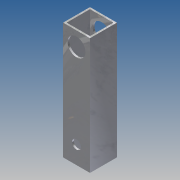
# Autodesk Inventor part: Z_Stage_Nut_holder_15x15alu
Saved by Autodesk Inventor 2015 SP1 (Build 190203100, 203)
## iProperties
Created: 2015-03-05
Part Number: Z_Stage_Nut_holder_15x15alu
Material: Aluminium 6061
Document SubType Name: Modeling
Designer: Marc
Density: 2.7 g/cm^3
Appearance: Aluminium - flach
Mass: 9.29786 g
Surface Area: 70.9355 cm^2
Volume: 3.44365 cm^3
Author: Marc
Autodesk Inventor part; units mm, degrees
ref_plane "YZ Plane" through (0, 0, 0) normal (1, 0, 0) x (0, 1, 0)
ref_plane "XZ Plane" through (0, 0, 0) normal (0, 1, 0) x (-1, 0, 0)
ref_plane "XY Plane" through (0, 0, 0) normal (0, 0, 1) x (1, 0, 0)
sketch "Skizze1" plane through (0, 0, 0) normal (0, 0, 1) x (1, 0, 0)
  line L0 (-10.5, 0) -> (10.5, 0) projected
  line L1 (0, -10.5) -> (0, 10.5) projected
  line L2 (-7.5, -7.5) -> (7.5, -7.5)
  line L3 (7.5, -7.5) -> (7.5, 7.5)
  line L4 (7.5, 7.5) -> (-7.5, 7.5)
  line L5 (-7.5, 7.5) -> (-7.5, -7.5)
  line L6 (-6.5, -6.5) -> (6.5, -6.5)
  line L7 (6.5, -6.5) -> (6.5, 6.5)
  line L8 (6.5, 6.5) -> (-6.5, 6.5)
  line L9 (-6.5, 6.5) -> (-6.5, -6.5)
  line L10 (-6.5, -6.5) -> (6.5, 6.5) construction
  line L11 (6.5, -6.5) -> (-6.5, 6.5) construction
  point P0 (0, 0)
  dimension "d0" = 15
  dimension "d1" = 15
  dimension "d2" = 13
  dimension "d3" = 13
  constraints: 20 end point, 4 parallel, 2 horizontal, 2 midpoint, 2 perpendicular, 2 other
  measures "d0" distance of L4.end L3.end
  measures "d1" distance of L3.end L2.end
  measures "d2" distance of L8.end L7.end
  measures "d3" distance of L7.end L6.end
extrude "Extrusion1" add sketch "Skizze1" along normal blind 65 contours L5 L4 L1 L8 L9 L0 | L0 L9 L6 L1 L2 L5 | L4 L3 L0 L7 L8 L1 | L1 L6 L7 L0 L3 L2
sketch "Skizze2" plane through (-7.5, 7.5, 0) normal (0, 1, 0) x (1, 0, 0)
  line L0 (15, 0) -> (0, 0) projected
  line L1 (0, 0) -> (0, -65) projected
  line L2 (15, -65) -> (0, -65) projected
  line L3 (15, 0) -> (15, -65) projected
  circle A0 centre (7.5, -57) radius 5
  circle A1 centre (7.5, -10) radius 2.5
  point P0 (7.5, 0)
  dimension "d6" = 10
  dimension "d7" = 8
  dimension "d8" = 7.5
  dimension "d9" = 5
  dimension "d10" = 7.5
  dimension "d11" = 10
  constraints: 2 centre point
  measures "d6" diameter of A0
  measures "d7" distance from line of L2 A0.centre
  measures "d8" distance from line of L3 A0.centre
  measures "d9" diameter of A1
  measures "d10" distance from line of L3 A1.centre
  measures "d11" distance from line of L0 A1.centre
extrude "Extrusion2" cut sketch "Skizze2" against normal blind 15 contours A0 | A1
equation "\"d10\" = d8"
